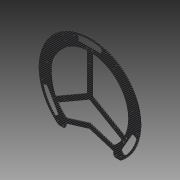
# Autodesk Inventor part: Middle Plate
Saved by Autodesk Inventor 2015 (Build 190159000, 159)
## iProperties
Created: 2016-08-09
Part Number: Middle Plate
Material: Generic
Document SubType Name: Modeling
Designer: James Yelland
Density: 1 g/cm^3
Appearance: Default
Author: James Yelland
Autodesk Inventor part; units mm, degrees
ref_plane "YZ Plane" through (0, 0, 0) normal (1, 0, 0) x (0, 1, 0)
ref_plane "XZ Plane" through (0, 0, 0) normal (0, 1, 0) x (-1, 0, 0)
ref_plane "XY Plane" through (0, 0, 0) normal (0, 0, 1) x (1, 0, 0)
sketch "Sketch1" plane through (0, 0, 0) normal (0, 1, 0) x (-1, 0, 0)
  line L0 (-62.9285, -83) -> (-54.3117, -83)
  line L1 (62.9285, -83) -> (54.3117, -83)
  arc A0 (65.4207, -82.1287) -> (-65.4207, -82.1287) centre (0, 0) ccw
  line L2 (-49.3117, -78) -> (-49.3117, -74.4821)
  line L3 (-47.8938, -72.5687) -> (0, -58)
  line L4 (49.3117, -78) -> (49.3117, -74.4821)
  line L5 (47.8938, -72.5687) -> (0, -58)
  arc A1 (49.3117, -78) -> (54.3117, -83) centre (54.3117, -78) ccw
  arc A2 (-54.3117, -83) -> (-49.3117, -78) centre (-54.3117, -78) ccw
  arc A3 (49.3117, -74.4821) -> (47.8938, -72.5687) centre (47.3117, -74.4821) ccw
  arc A4 (-47.8938, -72.5687) -> (-49.3117, -74.4821) centre (-47.3117, -74.4821) ccw
  arc A5 (62.9285, -83) -> (65.4207, -82.1287) centre (62.9285, -79) ccw
  arc A6 (-65.4207, -82.1287) -> (-62.9285, -83) centre (-62.9285, -79) ccw
  line L6 (-76.2102, -44) -> (-65.7102, -62.1865)
  line L7 (-67.1743, -67.6506) -> (-69.6351, -69.0713)
  line L8 (-94.6351, -25.7701) -> (-92.1743, -24.3494)
  line L9 (-86.7102, -25.8135) -> (-76.2102, -44)
  arc A7 (-96.4496, -30.438) -> (-74.5849, -68.3088) centre (0, 0) ccw
  arc A8 (-94.6351, -25.7701) -> (-96.4496, -30.438) centre (-92.6351, -29.2342) ccw
  arc A9 (-86.7102, -25.8135) -> (-92.1743, -24.3494) centre (-90.1743, -27.8135) ccw
  arc A10 (-67.1743, -67.6506) -> (-65.7102, -62.1865) centre (-69.1743, -64.1865) ccw
  arc A11 (-74.5849, -68.3088) -> (-69.6351, -69.0713) centre (-71.6351, -65.6072) ccw
  line L10 (65.7102, -62.1865) -> (76.2102, -44)
  arc A12 (74.5849, -68.3088) -> (96.4496, -30.438) centre (0, 0) ccw
  arc A13 (65.7102, -62.1865) -> (67.1743, -67.6506) centre (69.1743, -64.1865) ccw
  line L11 (69.6351, -69.0713) -> (67.1743, -67.6506)
  arc A14 (69.6351, -69.0713) -> (74.5849, -68.3088) centre (71.6351, -65.6072) ccw
  arc A15 (92.1743, -24.3494) -> (86.7102, -25.8135) centre (90.1743, -27.8135) ccw
  line L12 (92.1743, -24.3494) -> (94.6351, -25.7701)
  arc A16 (96.4496, -30.438) -> (94.6351, -25.7701) centre (92.6351, -29.2342) ccw
  line L13 (76.2102, -44) -> (86.7102, -25.8135)
  line L14 (21, 88) -> (0, 88)
  arc A17 (21.8647, 98.7468) -> (-21.8647, 98.7468) centre (0, 0) ccw
  arc A18 (21, 88) -> (25, 92) centre (21, 92) ccw
  line L15 (25, 94.8414) -> (25, 92)
  arc A19 (25, 94.8414) -> (21.8647, 98.7468) centre (21, 94.8414) ccw
  arc A20 (-25, 92) -> (-21, 88) centre (-21, 92) ccw
  line L16 (-25, 92) -> (-25, 94.8414)
  arc A21 (-21.8647, 98.7468) -> (-25, 94.8414) centre (-21, 94.8414) ccw
  line L17 (0, 88) -> (-21, 88)
  circle A22 centre (-33, 93.4207) radius 1.6
  circle A23 centre (33, 93.4207) radius 1.6
  line L18 (-75.1122, -39.9019) -> (-77.6122, -35.5718)
  line L19 (-77.6122, -35.5718) -> (-75.8801, -34.5718)
  line L20 (-75.8801, -34.5718) -> (-73.3801, -38.9019)
  line L21 (-73.3801, -38.9019) -> (-75.1122, -39.9019)
  line L22 (-70.3801, -44.0981) -> (-72.1122, -45.0981)
  line L23 (-67.8801, -48.4282) -> (-70.3801, -44.0981)
  line L24 (-69.6122, -49.4282) -> (-67.8801, -48.4282)
  line L25 (-72.1122, -45.0981) -> (-69.6122, -49.4282)
  line L26 (70.3801, -44.0981) -> (72.1122, -45.0981)
  line L27 (72.1122, -45.0981) -> (69.6122, -49.4282)
  line L28 (67.8801, -48.4282) -> (70.3801, -44.0981)
  line L29 (69.6122, -49.4282) -> (67.8801, -48.4282)
  line L30 (75.8801, -34.5718) -> (73.3801, -38.9019)
  line L31 (75.1122, -39.9019) -> (77.6122, -35.5718)
  line L32 (73.3801, -38.9019) -> (75.1122, -39.9019)
  line L33 (77.6122, -35.5718) -> (75.8801, -34.5718)
  line L34 (3, 83) -> (3, 85)
  line L35 (3, 85) -> (8, 85)
  line L36 (8, 83) -> (3, 83)
  line L37 (8, 85) -> (8, 83)
  line L38 (-8, 83) -> (-3, 83)
  line L39 (-3, 85) -> (-8, 85)
  line L40 (-3, 83) -> (-3, 85)
  line L41 (-8, 85) -> (-8, 83)
  circle A24 centre (-64.4047, -75.2892) radius 1.6
  circle A25 centre (-97.4047, -18.1315) radius 1.6
  circle A26 centre (97.4047, -18.1315) radius 1.6
  circle A27 centre (64.4047, -75.2892) radius 1.6
  line L42 (76.2102, -44) -> (69.282, -40)
  line L43 (0.597, -48.1867) -> (46.3795, -62.5064)
  line L44 (-0.597, -48.1867) -> (-46.3795, -62.5064)
  arc A28 (-51.0636, -61.5834) -> (-46.3795, -62.5064) centre (-47.8721, -57.7344) ccw
  arc A29 (0.597, -48.1867) -> (-0.597, -48.1867) centre (0, -50.0955) ccw
  arc A30 (46.3795, -62.5064) -> (51.0636, -61.5834) centre (47.8721, -57.7344) ccw
  line L45 (-5, 4.0415) -> (-5, 77.6853)
  line L46 (-69.7774, -34.5125) -> (-6, 2.3094)
  line L47 (5, 4.0415) -> (5, 77.6853)
  line L48 (6, 2.3094) -> (69.7774, -34.5125)
  line L49 (64.7774, -43.1728) -> (1, -6.3509)
  line L50 (-64.7774, -43.1728) -> (-1, -6.3509)
  arc A31 (-7.1795, 79.6772) -> (-72.5922, -33.621) centre (0, 0) ccw
  arc A32 (72.5922, -33.621) -> (7.1795, 79.6772) centre (0, 0) ccw
  arc A33 (51.0636, -61.5834) -> (65.4127, -46.0562) centre (0, 0) ccw
  arc A34 (-65.4127, -46.0562) -> (-51.0636, -61.5834) centre (0, 0) ccw
  circle A35 centre (-51.9527, -30.0153) radius 1.6
  circle A36 centre (0, 60) radius 1.6
  circle A37 centre (51.9527, -30.0153) radius 1.6
  arc A38 (69.7774, -34.5125) -> (72.5922, -33.621) centre (70.7774, -32.7805) ccw
  arc A39 (65.4127, -46.0562) -> (64.7774, -43.1728) centre (63.7774, -44.9048) ccw
  arc A40 (-64.7774, -43.1728) -> (-65.4127, -46.0562) centre (-63.7774, -44.9048) ccw
  arc A41 (-72.5922, -33.621) -> (-69.7774, -34.5125) centre (-70.7774, -32.7805) ccw
  arc A42 (-5, 77.6853) -> (-7.1795, 79.6772) centre (-7, 77.6853) ccw
  arc A43 (7.1795, 79.6772) -> (5, 77.6853) centre (7, 77.6853) ccw
  arc A44 (5, 4.0415) -> (6, 2.3094) centre (7, 4.0415) ccw
  arc A45 (-6, 2.3094) -> (-5, 4.0415) centre (-7, 4.0415) ccw
  arc A46 (1, -6.3509) -> (-1, -6.3509) centre (0, -8.0829) ccw
  circle A47 centre (50.0013, 74.8323) radius 1.6
  circle A48 centre (-50.0013, 74.8323) radius 1.6
  circle A49 centre (-88.2707, 17.5581) radius 1.6
  circle A50 centre (88.2707, 17.5581) radius 1.6
  line L51 (0, 0) -> (100, 0) construction
  line L52 (0, 0) -> (100, 0) construction
  circle A51 centre (55.557, 83.147) radius 1.6
  circle A52 centre (-55.557, 83.147) radius 1.6
  circle A53 centre (54.3117, -78) radius 1.6
  circle A54 centre (-54.3117, -78) radius 1.6
  point P0 (64.3117, -83)
  point P1 (-64.3117, -83)
  point P2 (-49.3117, -83)
  point P3 (49.3117, -83)
  point P4 (-49.3117, -73)
  point P5 (49.3117, -73)
  point P6 (-63.7102, -65.6506)
  point P7 (-72.3705, -70.6506)
  point P8 (-97.3705, -27.3494)
  point P9 (88.7102, -22.3494)
  point P10 (97.3705, -27.3494)
  point P11 (-25, 88)
  point P12 (-25, 98)
  point P13 (0, -48)
  point P14 (48.9186, -63.3006)
  point P15 (-48.9186, -63.3006)
  point P16 (-5, 79.8436)
  point P17 (5, 79.8436)
  point P18 (-66.6466, -44.2519)
  point P19 (-71.6466, -35.5917)
  point P20 (71.6466, -35.5917)
  point P21 (66.6466, -44.2519)
  point P22 (-5, 2.8868)
  point P23 (5, 2.8868)
  point P24 (0, -5.7735)
  dimension "d45" = 360
  dimension "d46" = 360
  dimension "d43" = 3.2
  dimension "d44" = 3.2
  dimension "d47" = 8
  dimension "d48" = 90
  dimension "d49" = 10
  dimension "d50" = 5
  dimension "d68" = 3.2
  dimension "d69" = 3.2
  dimension "d70" = 3.2
  dimension "d89" = 2
  dimension "d102" = 3.2
  dimension "d105" = 3.2
  dimension "d106" = 3.2
  dimension "d111" = 3.2
  dimension "d112" = 3.2
  dimension "d113" = 3.2
  constraints: 106 end point, 88 point on circle, 55 centre point, 36 point on line, 18 tangent, 8 coincident, 8 equal radius, 2 horizontal, 1 parallel, 2 other
  measures "d43" diameter of A22
  measures "d44" diameter of A23
  measures "d47" distance of L13.start L42.end
  measures "d48" angle of L10 L42
  measures "d49" distance of L5.end point (0, -48)
  measures "d50" radius of A28
  measures "d68" diameter of A35
  measures "d69" diameter of A36
  measures "d70" diameter of A37
  measures "d89" radius of A38
  measures "d102" diameter of A48
  measures "d105" diameter of A49
  measures "d106" diameter of A50
  measures "d111" diameter of A51
  measures "d112" diameter of A53
  measures "d113" diameter of A54
extrude "Extrusion1" add sketch "Sketch1" along normal blind 2
body "Solid1"
